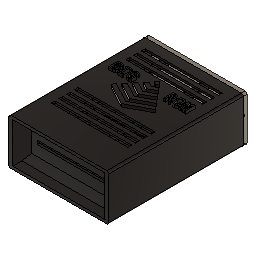
case (Autodesk Fusion 360 design; units mm, degrees)
Autodesk Fusion 360 part; units mm, degrees
note: some values were not read from the file. Chosen so that the rebuilt part matches the saved one: which bodies a step acts on.
(part 1 of 3)
sketch "Schizzo1" plane through (0, 0, 0) normal (0, 0, 1) x (1, 0, 0)
  line L0 (0, 0) -> (52, 0)
  line L1 (52, 0) -> (52, 70)
  line L2 (52, 70) -> (0, 70)
  line L3 (0, 70) -> (0, 0)
  dimension "d1" = 52
  dimension "d2" = 70
  constraint horizontal L0
  constraint vertical L1
  constraint horizontal L2
  constraint vertical L3
  constraint coincident L0.start L3.end
  measures "d1" distance of L0.start L0.end
  measures "d2" distance of L0.start L2.end
extrude "Estrusione1" add sketch "Schizzo1" along normal blind 24 makes body 1
sketch "Schizzo2" plane through (0, 0, 0) normal (0, -1, 0) x (1, 0, 0)
  line L0 (0, 0) -> (52, 0)
  line L1 (52, 0) -> (52, 24)
  line L2 (52, 24) -> (0, 24)
  line L3 (0, 24) -> (0, 0)
  line L4 (2, 22.5) -> (50, 22.5)
  line L5 (50, 22.5) -> (50, 1.5)
  line L6 (50, 1.5) -> (2, 1.5)
  line L7 (2, 1.5) -> (2, 22.5)
  dimension "d5" = 2
  dimension "d6" = 1.5
  dimension "d7" = 1.5
  dimension "d8" = 2
  constraint horizontal L4
  constraint vertical L5
  constraint horizontal L6
  constraint vertical L7
  measures "d5" horizontal distance of L2.end L4.start
  measures "d6" vertical distance of L2.end L4.start
  measures "d7" vertical distance of L0.start L6.end
  measures "d8" horizontal distance of L0.end L5.end
extrude "Estrusione2" cut sketch "Schizzo2" against normal blind 9.8 contours L4 L5 L6 L7 bodies 1
sketch "Schizzo3" plane through (0, 70, 0) normal (0, 1, 0) x (-1, 0, 0)
  line L0 (-52, 0) -> (0, 0)
  line L1 (0, 0) -> (0, 24)
  line L2 (0, 24) -> (-52, 24)
  line L3 (-52, 24) -> (-52, 0)
  line L4 (-48, 1) -> (-48, 8)
  line L5 (-48, 8) -> (-50.25, 8)
  line L6 (-50.25, 8) -> (-50.25, 9.7)
  line L7 (-50.25, 9.7) -> (-48, 9.7)
  line L8 (-48, 9.7) -> (-48, 23)
  line L9 (-48, 23) -> (-4, 23)
  line L10 (-4, 23) -> (-4, 9.7)
  line L11 (-4, 9.7) -> (-1.75, 9.7)
  line L12 (-1.75, 9.7) -> (-1.75, 8)
  line L13 (-1.75, 8) -> (-4, 8)
  line L14 (-4, 8) -> (-4, 1)
  line L15 (-4, 1) -> (-48, 1)
  dimension "d11" = 2.25
  dimension "d12" = 1.7
  dimension "d13" = 2.25
  dimension "d14" = 1
  dimension "d15" = 4
  dimension "d16" = 4
  dimension "d17" = 1
  dimension "d62" = 8
  constraint vertical L4
  constraint perpendicular L4 L5
  constraint perpendicular L5 L6
  constraint perpendicular L6 L7
  constraint perpendicular L7 L8
  constraint perpendicular L6 L9
  constraint perpendicular L9 L10
  constraint perpendicular L10 L11
  constraint perpendicular L11 L12
  constraint perpendicular L12 L13
  constraint perpendicular L13 L14
  constraint perpendicular L4 L15
  constraint equal L8 L10
  constraint equal L5 L7
  constraint equal L11 L13
  constraint equal L6 L12
  measures "d11" distance of L4.end L5.end
  measures "d12" distance of L5.end L6.end
  measures "d13" distance of L10.end L11.end
  measures "d14" vertical distance of L2.end L8.end
  measures "d15" horizontal distance of L0.start L4.start
  measures "d16" horizontal distance of L0.end L14.end
  measures "d17" vertical distance of L0.end L14.end
  measures "d62" vertical distance of L0.start L4.end
extrude "Estrusione3" cut sketch "Schizzo3" against normal blind 59 contours L4 L5 L6 L7 L8 L9 L10 L11 L12 L13 L14 L15 bodies 1
sketch "Schizzo4" plane through (0, 11, 0) normal (0, 1, 0) x (-1, 0, 0)
  line L0 (-4, 1) -> (-4, 8)
  line L1 (-4, 8) -> (-1.75, 8)
  line L2 (-1.75, 8) -> (-1.75, 9.7)
  line L3 (-1.75, 9.7) -> (-4, 9.7)
  line L4 (-4, 9.7) -> (-4, 23)
  line L5 (-4, 23) -> (-48, 23)
  line L6 (-48, 23) -> (-48, 9.7)
  line L7 (-48, 9.7) -> (-50.25, 9.7)
  line L8 (-50.25, 9.7) -> (-50.25, 8)
  line L9 (-50.25, 8) -> (-48, 8)
  line L10 (-48, 8) -> (-48, 1)
  line L11 (-48, 1) -> (-4, 1)
  line L12 (-47, 9.85) -> (-5, 9.85)
  line L13 (-5, 9.85) -> (-5, 7.85)
  line L14 (-5, 7.85) -> (-47, 7.85)
  line L15 (-47, 7.85) -> (-47, 9.85)
  line L16 (-26, 23) -> (-26, 1) construction
  line L17 (-50.25, 8.85) -> (-1.75, 8.85) construction
  dimension "d20" = 42
  dimension "d21" = 2
  constraint horizontal L12
  constraint vertical L13
  constraint horizontal L14
  constraint vertical L15
  constraint midpoint L5 L16.start
  constraint midpoint L11 L16.end
  constraint midpoint L8 L17.start
  constraint midpoint L2 L17.end
  constraint symmetric L13.end L14.end L16
  constraint symmetric L12.start L14.end L17
  measures "d20" distance of L12.start L12.end
  measures "d21" distance of L12.start L14.end
extrude "Estrusione4" cut sketch "Schizzo4" against normal through all contours L12 L13 L14 L15 bodies 1
sketch "Schizzo5" plane through (0, 0, 24) normal (0, 0, 1) x (-1, 0, 0)
  line L0 (0, -70) -> (0, 0)
  line L1 (0, 0) -> (-52, 0)
  line L2 (-52, -70) -> (0, -70)
  line L3 (-6, -55) -> (-46, -55)
  line L4 (-6, -30) -> (-46, -30)
  line L5 (-6, -55) -> (-6, -57)
  line L6 (-6, -57) -> (-46, -57)
  line L7 (-46, -57) -> (-46, -55)
  line L8 (-6, -30) -> (-6, -28)
  line L9 (-6, -28) -> (-46, -28)
  line L10 (-46, -28) -> (-46, -30)
  line L11 (-6, -59) -> (-46, -59)
  line L12 (-46, -59) -> (-46, -61)
  line L13 (-46, -61) -> (-6, -61)
  line L14 (-6, -61) -> (-6, -59)
  line L15 (-6, -63) -> (-46, -63)
  line L16 (-46, -63) -> (-46, -65)
  line L17 (-46, -65) -> (-6, -65)
  line L18 (-6, -65) -> (-6, -63)
  line L19 (-6, -26) -> (-46, -26)
  line L20 (-46, -26) -> (-46, -24)
  line L21 (-46, -24) -> (-6, -24)
  line L22 (-6, -24) -> (-6, -26)
  line L23 (-6, -22) -> (-46, -22)
  line L24 (-46, -22) -> (-46, -20)
  line L25 (-46, -20) -> (-6, -20)
  line L26 (-6, -20) -> (-6, -22)
  line L27 (-6, -18) -> (-46, -18)
  line L28 (-46, -18) -> (-46, -16)
  line L29 (-46, -16) -> (-6, -16)
  line L30 (-6, -16) -> (-6, -18)
  dimension "d34" = 25
  dimension "d146" = 40
  dimension "d147" = 2
  dimension "d148" = 40
  dimension "d149" = 2
  dimension "d150" = 40
  dimension "d151" = 2
  dimension "d152" = 40
  dimension "d153" = 2
  dimension "d154" = 40
  dimension "d155" = 2
  dimension "d156" = 2
  dimension "d157" = 2
  dimension "d158" = 2
  dimension "d159" = 5
  dimension "d160" = 6
  dimension "d162" = 40
  dimension "d163" = 40
  dimension "d164" = 2
  dimension "d165" = 2
  dimension "d166" = 2
  dimension "d167" = 6
  dimension "d168" = 16
  constraint horizontal L4
  constraint equal L3 L4
  constraint perpendicular L3 L5
  constraint perpendicular L5 L6
  constraint perpendicular L4 L8
  constraint perpendicular L8 L9
  constraint horizontal L11
  constraint vertical L12
  constraint horizontal L13
  constraint vertical L14
  constraint horizontal L15
  constraint vertical L16
  constraint horizontal L17
  constraint vertical L18
  constraint horizontal L19
  constraint vertical L20
  constraint horizontal L21
  constraint vertical L22
  constraint horizontal L23
  constraint vertical L24
  constraint horizontal L25
  constraint vertical L26
  constraint horizontal L27
  constraint vertical L28
  constraint horizontal L29
  constraint vertical L30
  constraint equal L4 L9
  constraint vertical L25.end L27.start
  constraint vertical L21.end L23.start
  measures "d34" distance of L3.start L4.start
  measures "d146" distance of L11.start L11.end
  measures "d147" distance of L11.start L13.end
  measures "d148" distance of L15.start L15.end
  measures "d149" distance of L15.start L17.end
  measures "d150" distance of L19.start L19.end
  measures "d151" distance of L19.start L21.end
  measures "d152" distance of L23.start L23.end
  measures "d153" distance of L23.start L25.end
  measures "d154" distance of L27.start L27.end
  measures "d155" distance of L27.start L29.end
  measures "d156" distance of L3.start L5.end
  measures "d157" distance of L5.end L11.start
  measures "d158" distance of L13.end L15.start
  measures "d159" vertical distance of L0.start L17.end
  measures "d160" horizontal distance of L0.start L17.end
  measures "d162" distance of L5.end L6.end
  measures "d163" distance of L3.start L3.end
  measures "d164" distance of L8.end L19.start
  measures "d165" distance of L21.end L23.start
  measures "d166" distance of L25.end L27.start
  measures "d167" horizontal distance of L0.end L29.end
  measures "d168" vertical distance of L1.end L28.end
extrude "Estrusione5" cut sketch "Schizzo5" against normal blind 2 bodies 1
sketch "Schizzo6" plane through (0, 70, 0) normal (0, 1, 0) x (-1, 0, 0)
  line L0 (-1.75, 8) -> (-4, 8)
  line L1 (-4, 8) -> (-4, 1)
  line L2 (-4, 1) -> (-48, 1)
  line L3 (-48, 1) -> (-48, 8)
  line L4 (-48, 8) -> (-50.25, 8)
  line L5 (-50.25, 8) -> (-50.25, 9.7)
  line L6 (-50.25, 9.7) -> (-48, 9.7)
  line L7 (-48, 9.7) -> (-48, 23)
  line L8 (-48, 23) -> (-4, 23)
  line L9 (-4, 23) -> (-4, 9.7)
  line L10 (-4, 9.7) -> (-1.75, 9.7)
  line L11 (-1.75, 9.7) -> (-1.75, 8)
  line L12 (-52, 0) -> (0, 0)
  line L13 (0, 0) -> (0, 24)
  line L14 (0, 24) -> (-52, 24)
  line L15 (-52, 24) -> (-52, 0)
  circle A0 centre (-50, 12.7) radius 1
  circle A1 centre (-2, 12.7) radius 1
  dimension "d44" = 2
  dimension "d45" = 2
  dimension "d46" = 2
  dimension "d47" = 2
  dimension "d121" = 3
  constraint horizontal A0.centre A1.centre
  measures "d44" horizontal distance of L14.end A0.centre
  measures "d45" diameter of A0
  measures "d46" diameter of A1
  measures "d47" horizontal distance of L13.end A1.centre
  measures "d121" vertical distance of L5.end A0.centre
hole "Foratura1" at (50, 70, 12.7) at (2, 70, 12.7) direction (0, -1, 0) diameter 1.3 depth 20 tip angle 118 bodies 1
sketch "Schizzo7" plane through (0, 0, 1) normal (0, 0, 1) x (-1, 0, 0)
  line L0 (-48, -70) -> (-4, -70)
  line L1 (-4, -70) -> (-4, -11)
  line L2 (-4, -11) -> (-48, -11)
  line L3 (-48, -11) -> (-48, -70)
  line L4 (-14, -11) -> (-14, -31)
  line L5 (-14, -31) -> (-4, -31)
  line L6 (-4, -46) -> (-14, -46)
  line L7 (-14, -46) -> (-14, -70)
  line L8 (-17, -70) -> (-17, -46)
  line L9 (-17, -46) -> (-35, -46)
  line L10 (-35, -46) -> (-35, -70)
  line L11 (-38, -70) -> (-38, -46)
  line L12 (-38, -46) -> (-48, -46)
  line L13 (-48, -31) -> (-38, -31)
  line L14 (-38, -31) -> (-38, -11)
  line L15 (-38, -11) -> (-35, -11)
  line L16 (-35, -31) -> (-17, -31)
  line L17 (-17, -31) -> (-17, -11)
  line L18 (-35, -31) -> (-35, -11)
  line L19 (-4, -46) -> (-4, -31)
  line L20 (-48, -46) -> (-48, -31)
  line L21 (-14, -11) -> (-17, -11)
  line L22 (-14, -70) -> (-17, -70)
  line L23 (-35, -70) -> (-38, -70)
  dimension "d52" = 20
  dimension "d53" = 3
  dimension "d54" = 10
  dimension "d55" = 15
  constraint coincident L2 L4.start
  constraint perpendicular L2 L4
  constraint coincident L1 L5.end
  constraint perpendicular L1 L5
  constraint coincident L1 L6.start
  constraint perpendicular L1 L6
  constraint coincident L0 L7.end
  constraint perpendicular L0 L7
  constraint coincident L0 L8.start
  constraint perpendicular L0 L8
  constraint perpendicular L8 L9
  constraint coincident L0 L10.end
  constraint perpendicular L0 L10
  constraint coincident L0 L11.start
  constraint perpendicular L0 L11
  constraint coincident L3 L12.end
  constraint perpendicular L3 L12
  constraint coincident L3 L13.start
  constraint perpendicular L3 L13
  constraint coincident L2 L14.end
  constraint perpendicular L2 L14
  constraint coincident L2 L15.end
  constraint perpendicular L3 L15
  constraint parallel L15 L16
  constraint coincident L2 L17.end
  constraint perpendicular L16 L17
  constraint perpendicular L15 L18
  constraint equal L15 L21
  constraint equal L22 L23
  constraint equal L21 L22
  constraint equal L19 L20
  constraint equal L14 L18
  constraint equal L4 L18
  constraint equal L7 L8
  constraint equal L5 L6
  constraint equal L9 L16
  constraint equal L5 L13
  measures "d52" distance of L4.start L4.end
  measures "d53" distance of L4.start L17.end
  measures "d54" distance of L4.end L5.end
  measures "d55" distance of L5.end L6.start
extrude "Estrusione6" add sketch "Schizzo7" along normal blind 1.5 contours L0 L1 L2 L3 L4 L5 L6 L7 L8 L9 L10 L11 L12 L13 L14 L15 L16 L17 L18 L19 L20 L21 L22 L23 bodies 1
ref_plane "Piano di lavoro2" through (0, 0, 23) normal (0, 0, 1) x (1, 0, 0)
sketch "Schizzo10" plane through (0, 0, 23) normal (0, 0, 1) x (1, 0, 0)
  line L0 (38, 70) -> (38, 50)
  line L1 (38, 50) -> (48, 50)
  line L2 (48, 50) -> (48, 35)
  line L3 (48, 35) -> (38, 35)
  line L4 (38, 35) -> (38, 11)
  line L5 (38, 11) -> (35, 11)
  line L6 (35, 11) -> (35, 35)
  line L7 (35, 35) -> (17, 35)
  line L8 (17, 35) -> (17, 11)
  line L9 (17, 11) -> (14, 11)
  line L10 (14, 11) -> (14, 35)
  line L11 (14, 35) -> (4, 35)
  line L12 (4, 35) -> (4, 50)
  line L13 (4, 50) -> (14, 50)
  line L14 (14, 50) -> (14, 70)
  line L15 (14, 70) -> (17, 70)
  line L16 (17, 70) -> (17, 50)
  line L17 (17, 50) -> (35, 50)
  line L18 (35, 50) -> (35, 70)
  line L19 (35, 70) -> (38, 70)
  line L20 (48, 70) -> (4, 70)
  line L21 (48, 11) -> (4, 11)
  dimension "d65" = 3
  dimension "d66" = 15
  dimension "d67" = 20
  dimension "d68" = 10
  constraint vertical L0
  constraint perpendicular L0 L1
  constraint perpendicular L1 L2
  constraint perpendicular L2 L3
  constraint perpendicular L1 L4
  constraint perpendicular L4 L5
  constraint perpendicular L5 L6
  constraint perpendicular L6 L7
  constraint perpendicular L5 L8
  constraint perpendicular L8 L9
  constraint perpendicular L9 L10
  constraint perpendicular L10 L11
  constraint perpendicular L11 L12
  constraint perpendicular L12 L13
  constraint perpendicular L11 L14
  constraint perpendicular L14 L15
  constraint perpendicular L15 L16
  constraint perpendicular L16 L17
  constraint perpendicular L15 L18
  constraint perpendicular L0 L19
  constraint equal L5 L19
  constraint equal L9 L15
  constraint equal L5 L9
  constraint equal L0 L18
  constraint equal L16 L18
  constraint equal L14 L16
  constraint equal L8 L10
  constraint equal L4 L6
  constraint equal L1 L3
  constraint equal L7 L17
  constraint coincident L18.end L20
  constraint coincident L5.end L21
  constraint equal L1 L13
  constraint coincident L8.end L21
  constraint vertical L11.end L21.end
  constraint vertical L2.end L21.start
  measures "d65" distance of L0.start L18.end
  measures "d66" distance of L1.end L2.end
  measures "d67" distance of L0.start L0.end
  measures "d68" distance of L0.end L1.end
extrude "Estrusione7" add sketch "Schizzo10" against normal blind 1.5 contours L0 L1 L2 L3 L4 L5 L6 L7 L8 L9 L10 L11 L12 L13 L14 L15 L16 L17 L18 L19 L20 L21 bodies 1
sketch "Schizzo11" plane through (0, 0, 24) normal (0, 0, 1) x (-1, 0, 0)
  line L0 (-6, -30) -> (-46, -30)
  line L1 (-46, -55) -> (-6, -55)
  line L2 (0, -70) -> (0, 0)
  line L3 (0, 0) -> (-52, 0)
  line L4 (-52, 0) -> (-52, -70)
  line L5 (-52, -70) -> (0, -70)
  line L6 (-6, -50.9797) -> (-7.5273, -50.9797)
  spline S0 degree 2 poles (-7.5273, -50.9797) (-8.4582, -50.9797) (-8.8924, -50.6722) knots 0 0 0 1 1 1
  spline S1 degree 2 poles (-8.8924, -50.6722) (-9.3266, -50.3647) (-9.3266, -49.685) knots 0 0 0 1 1 1
  spline S2 degree 2 poles (-9.3266, -49.685) (-9.3266, -49.2344) (-9.0486, -48.9336) knots 0 0 0 1 1 1
  spline S3 degree 2 poles (-9.4618, -47.4715) (-9.4618, -46.7868) (-9.0172, -46.3934) knots 0 0 0 1 1 1
  spline S4 degree 2 poles (-9.0172, -46.3934) (-8.5725, -46) (-7.8154, -46) knots 0 0 0 1 1 1
  line L7 (-7.8154, -46) -> (-6, -46)
  line L8 (-6, -46) -> (-6, -50.9797)
  line L9 (-6.7552, -48.9277) -> (-7.6187, -48.9277)
  spline S5 degree 2 poles (-7.6187, -48.9277) (-8.1089, -48.9277) (-8.3219, -49.0924) knots 0 0 0 1 1 1
  spline S6 degree 2 poles (-8.3219, -49.0924) (-8.535, -49.2572) (-8.535, -49.6441) knots 0 0 0 1 1 1
  spline S7 degree 2 poles (-8.535, -49.6441) (-8.535, -50.0046) (-8.306, -50.161) knots 0 0 0 1 1 1
  spline S8 degree 2 poles (-8.306, -50.161) (-8.077, -50.3175) (-7.5529, -50.3175) knots 0 0 0 1 1 1
  line L10 (-7.5529, -50.3175) -> (-6.7552, -50.3175)
  line L11 (-6.7552, -50.3175) -> (-6.7552, -48.9277)
  line L12 (-6.7552, -48.2654) -> (-6.7552, -46.6622)
  line L13 (-6.7552, -46.6622) -> (-7.7043, -46.6622)
  spline S9 degree 2 poles (-7.7043, -46.6622) (-8.6702, -46.6622) (-8.6702, -47.4967) knots 0 0 0 1 1 1
  spline S10 degree 2 poles (-8.6702, -47.4967) (-8.6702, -48.2654) (-7.6611, -48.2654) knots 0 0 0 1 1 1
  line L14 (-7.6611, -48.2654) -> (-6.7552, -48.2654)
  line L15 (-13.1262, -46) -> (-10.4187, -46)
  line L16 (-10.4187, -46) -> (-10.4187, -46.5376)
  line L17 (-10.4187, -46.5376) -> (-11.3966, -46.6039)
  line L18 (-11.3966, -46.6039) -> (-11.3966, -50.3747)
  line L19 (-11.3966, -50.3747) -> (-10.4187, -50.441)
  line L20 (-10.4187, -50.441) -> (-10.4187, -50.9797)
  line L21 (-10.4187, -50.9797) -> (-13.1262, -50.9797)
  line L22 (-13.1262, -50.9797) -> (-13.1262, -50.4413)
  line L23 (-13.1262, -50.4413) -> (-12.1517, -50.3751)
  line L24 (-12.1517, -50.3751) -> (-12.1517, -46.6036)
  line L25 (-12.1517, -46.6036) -> (-13.1262, -46.5373)
  line L26 (-13.1262, -46.5373) -> (-13.1262, -46)
  line L27 (-16.0196, -48.6944) -> (-17.5571, -48.6944)
  line L28 (-17.5571, -48.6944) -> (-17.5571, -46.2033)
  spline S11 degree 2 poles (-17.5571, -46.2033) (-16.8532, -45.9324) (-16.0939, -45.9324) knots 0 0 0 1 1 1
  spline S12 degree 2 poles (-16.0939, -45.9324) (-15.19, -45.9324) (-14.6849, -46.6156) knots 0 0 0 1 1 1
  spline S13 degree 2 poles (-14.6849, -46.6156) (-14.1799, -47.2988) (-14.1799, -48.4965) knots 0 0 0 1 1 1
  spline S14 degree 2 poles (-14.1799, -48.4965) (-14.1799, -49.6843) (-14.7346, -50.3675) knots 0 0 0 1 1 1
  spline S15 degree 2 poles (-14.7346, -50.3675) (-15.2893, -51.0507) (-16.2629, -51.0507) knots 0 0 0 1 1 1
  spline S16 degree 2 poles (-16.2629, -51.0507) (-16.9168, -51.0507) (-17.4809, -50.7257) knots 0 0 0 1 1 1
  line L29 (-17.4809, -50.7257) -> (-17.2047, -50.0935)
  spline S17 degree 2 poles (-17.2047, -50.0935) (-16.669, -50.3719) (-16.2445, -50.3719) knots 0 0 0 1 1 1
  spline S18 degree 2 poles (-16.2445, -50.3719) (-15.647, -50.3719) (-15.3092, -49.8807) knots 0 0 0 1 1 1
  spline S19 degree 2 poles (-15.3092, -49.8807) (-14.9715, -49.3894) (-14.9715, -48.4915) knots 0 0 0 1 1 1
  spline S20 degree 2 poles (-14.9715, -48.4915) (-14.9715, -46.6112) (-16.2022, -46.6112) knots 0 0 0 1 1 1
  spline S21 degree 2 poles (-16.2022, -46.6112) (-16.5151, -46.6112) (-16.802, -46.6906) knots 0 0 0 1 1 1
  line L30 (-16.802, -46.6906) -> (-16.802, -48.0156)
  line L31 (-16.802, -48.0156) -> (-16.0196, -48.0156)
  line L32 (-16.0196, -48.0156) -> (-16.0196, -48.6944)
  spline S22 degree 2 poles (-9.0486, -48.9336) (-8.8398, -48.7075) (-8.5566, -48.6203) knots 0 0 0 0.751565 0.751565 0.751565
  spline S23 degree 2 poles (-8.5566, -48.6203) (-9.4618, -48.3879) (-9.4618, -47.4715) knots 0.093077 0.093077 0.093077 1 1 1
  line L33 (-35.2961, -47.9983) -> (-35.2961, -46)
  line L34 (-35.2961, -46) -> (-34.5409, -46)
  line L35 (-34.5409, -46) -> (-34.5409, -50.9797)
  line L36 (-34.5409, -50.9797) -> (-35.792, -50.9797)
  spline S24 degree 2 poles (-35.792, -50.9797) (-37.5869, -50.9797) (-37.5869, -49.5355) knots 0 0 0 1 1 1
  spline S25 degree 2 poles (-37.5869, -49.5355) (-37.5869, -48.5363) (-36.6274, -48.1996) knots 0 0 0 1 1 1
  line L37 (-36.6274, -48.1996) -> (-37.9461, -46)
  line L38 (-37.9461, -46) -> (-37.1091, -46)
  line L39 (-37.1091, -46) -> (-35.9453, -47.9983)
  line L40 (-35.9453, -47.9983) -> (-35.2961, -47.9983)
  line L41 (-35.2961, -48.6606) -> (-35.7655, -48.6606)
  spline S26 degree 2 poles (-35.7655, -48.6606) (-36.305, -48.6606) (-36.5502, -48.8613) knots 0 0 0 1 1 1
  spline S27 degree 2 poles (-36.5502, -48.8613) (-36.7953, -49.0621) (-36.7953, -49.5072) knots 0 0 0 1 1 1
  spline S28 degree 2 poles (-36.7953, -49.5072) (-36.7953, -49.9402) (-36.5531, -50.1288) knots 0 0 0 1 1 1
  spline S29 degree 2 poles (-36.5531, -50.1288) (-36.311, -50.3175) (-35.749, -50.3175) knots 0 0 0 1 1 1
  line L42 (-35.749, -50.3175) -> (-35.2961, -50.3175)
  line L43 (-35.2961, -50.3175) -> (-35.2961, -48.6606)
  spline S30 degree 2 poles (-40.1538, -45.9324) (-38.3215, -45.9324) (-38.3215, -48.5032) knots 0 0 0 1 1 1
  spline S31 degree 2 poles (-38.3215, -48.5032) (-38.3215, -51.0575) (-40.1604, -51.0575) knots 0 0 0 1 1 1
  spline S32 degree 2 poles (-40.1604, -51.0575) (-41.0466, -51.0575) (-41.5164, -50.385) knots 0 0 0 1 1 1
  spline S33 degree 2 poles (-41.5164, -50.385) (-41.9861, -49.7124) (-41.9861, -48.4966) knots 0 0 0 1 1 1
  spline S34 degree 2 poles (-41.9861, -48.4966) (-41.9861, -47.2795) (-41.5117, -46.606) knots 0 0 0 1 1 1
  spline S35 degree 2 poles (-41.5117, -46.606) (-41.0372, -45.9324) (-40.1538, -45.9324) knots 0 0 0 1 1 1
  spline S36 degree 2 poles (-40.1538, -46.6112) (-40.6881, -46.6112) (-40.9413, -47.0666) knots 0 0 0 1 1 1
  spline S37 degree 2 poles (-40.9413, -47.0666) (-41.1945, -47.5219) (-41.1945, -48.4983) knots 0 0 0 1 1 1
  spline S38 degree 2 poles (-41.1945, -48.4983) (-41.1945, -49.483) (-40.938, -49.9308) knots 0 0 0 1 1 1
  spline S39 degree 2 poles (-40.938, -49.9308) (-40.6815, -50.3786) (-40.1604, -50.3786) knots 0 0 0 1 1 1
  spline S40 degree 2 poles (-40.1604, -50.3786) (-39.1131, -50.3786) (-39.1131, -48.4983) knots 0 0 0 1 1 1
  spline S41 degree 2 poles (-39.1131, -48.4983) (-39.1131, -46.6112) (-40.1538, -46.6112) knots 0 0 0 1 1 1
  line L44 (-43.9423, -46) -> (-43.1615, -49.596)
  line L45 (-43.1806, -48.9646) -> (-43.1806, -46)
  line L46 (-43.1806, -46) -> (-42.5382, -46)
  line L47 (-42.5382, -46) -> (-42.5382, -50.9797)
  line L48 (-42.5382, -50.9797) -> (-43.4818, -50.9797)
  line L49 (-43.4818, -50.9797) -> (-44.2572, -47.2526)
  line L50 (-44.2572, -47.2526) -> (-45.0388, -50.9797)
  line L51 (-45.0388, -50.9797) -> (-46, -50.9797)
  line L52 (-46, -50.9797) -> (-46, -46)
  line L53 (-46, -46) -> (-45.3576, -46)
  line L54 (-45.3576, -46) -> (-45.3576, -49.0077)
  line L55 (-45.3766, -49.6687) -> (-44.5647, -46)
  line L56 (-44.5647, -46) -> (-43.9423, -46)
  spline S42 degree 2 poles (-43.1615, -49.596) (-43.1806, -49.2202) (-43.1806, -48.9646) knots 0.433911 0.433911 0.433911 1 1 1
  spline S43 degree 2 poles (-45.3576, -49.0077) (-45.3576, -49.2263) (-45.3766, -49.6687) knots 0 0 0 0.640385 0.640385 0.640385
  line L57 (-46, -28) -> (-6, -28)
  line L58 (-6, -28) -> (-6, -30)
  line L59 (-46, -30) -> (-46, -28)
  line L60 (-46, -57) -> (-46, -55)
  line L61 (-6, -55) -> (-6, -57)
  line L62 (-6, -57) -> (-46, -57)
  line L63 (-46, -18) -> (-46, -16)
  line L64 (-46, -16) -> (-6, -16)
  line L65 (-6, -16) -> (-6, -18)
  line L66 (-6, -18) -> (-46, -18)
  line L67 (-46, -22) -> (-46, -20)
  line L68 (-46, -20) -> (-6, -20)
  line L69 (-6, -20) -> (-6, -22)
  line L70 (-6, -22) -> (-46, -22)
  line L71 (-46, -59) -> (-6, -59)
  line L72 (-6, -59) -> (-6, -61)
  line L73 (-6, -61) -> (-46, -61)
  line L74 (-46, -61) -> (-46, -59)
  line L75 (-46, -26) -> (-46, -24)
  line L76 (-46, -24) -> (-6, -24)
  line L77 (-6, -24) -> (-6, -26)
  line L78 (-6, -26) -> (-46, -26)
  line L79 (-46, -63) -> (-6, -63)
  line L80 (-6, -63) -> (-6, -65)
  line L81 (-6, -65) -> (-46, -65)
  line L82 (-46, -65) -> (-46, -63)
extrude "Estrusione1'" add sketch "Schizzo11" along normal blind 1.5 separate body contours L6 S0 S1 S2 S3 S4 L7 L8 S22 S23 | L15 L16 L17 L18 L19 L20 L21 L22 L23 L24 L25 L26 | L27 L28 S11 S12 S13 S14 S15 S16 L29 S17 S18 S19 S20 S21 L30 L31 L32 | L33 L34 L35 L36 S24 S25 L37 L38 L39 L40 | S30 S31 S32 S33 S34 S35 | L44 L45 L46 L47 L48 L49 L50 L51 L52 L53 L54 L55 L56 S42 S43 makes body 2 at (11.9, 47.8609, 24) makes body 3 at (17.3054, 47.6377, 24) makes body 4 at (43.0605, 50.5185, 24) makes body 5 at (6.2517, 48.415, 24) makes body 6 at (38.6059, 48.8805, 24) makes body 7 at (34.7926, 48.5468, 24) in component "Componente_Testo"
sketch "Schizzo12" plane through (0, 0, 24) normal (0, 0, 1) x (-1, 0, 0)
  line L0 (-6, -30) -> (-46, -30)
  line L1 (-46, -55) -> (-6, -55)
  line L2 (0, -70) -> (0, 0)
  line L3 (0, 0) -> (-52, 0)
  line L4 (-52, 0) -> (-52, -70)
  line L5 (-52, -70) -> (0, -70)
  spline S0 degree 3 poles (-25.8442, -38.9932) (-25.6519, -39.0542) (-25.2683, -39.375) (-24.4958, -39.8248) knots 0 0 0 0 1 1 1 1
  line L6 (-25.8442, -38.9932) -> (-25.6519, -39.0542) construction
  line L7 (-25.6519, -39.0542) -> (-25.2683, -39.375) construction
  line L8 (-25.2683, -39.375) -> (-24.4958, -39.8248) construction
  spline S1 degree 3 poles (-24.4958, -39.8248) (-23.9962, -40.1158) (-23.6534, -40.3101) (-22.8266, -40.7709) knots 0 0 0 0 1 1 1 1
  line L9 (-24.4958, -39.8248) -> (-23.9962, -40.1158) construction
  line L10 (-23.9962, -40.1158) -> (-23.6534, -40.3101) construction
  line L11 (-23.6534, -40.3101) -> (-22.8266, -40.7709) construction
  spline S2 degree 3 poles (-22.8266, -40.7709) (-20.957, -41.8131) (-19.8024, -42.4728) (-19.2156, -42.8342) knots 0 0 0 0 1 1 1 1
  line L12 (-22.8266, -40.7709) -> (-20.957, -41.8131) construction
  line L13 (-20.957, -41.8131) -> (-19.8024, -42.4728) construction
  line L14 (-19.8024, -42.4728) -> (-19.2156, -42.8342) construction
  spline S3 degree 3 poles (-19.2156, -42.8342) (-19.0296, -42.9487) (-18.8671, -43.0807) (-18.8872, -43.1008) knots 0 0 0 0 1 1 1 1
  line L15 (-19.2156, -42.8342) -> (-19.0296, -42.9487) construction
  line L16 (-19.0296, -42.9487) -> (-18.8671, -43.0807) construction
  line L17 (-18.8671, -43.0807) -> (-18.8872, -43.1008) construction
  spline S4 degree 3 poles (-18.8872, -43.1008) (-18.9205, -43.1341) (-19.4317, -42.875) (-21.4715, -41.7912) knots 0 0 0 0 1 1 1 1
  line L18 (-18.8872, -43.1008) -> (-18.9205, -43.1341) construction
  line L19 (-18.9205, -43.1341) -> (-19.4317, -42.875) construction
  line L20 (-19.4317, -42.875) -> (-21.4715, -41.7912) construction
  spline S5 degree 3 poles (-21.4715, -41.7912) (-23.3012, -40.8189) (-23.623, -40.65) (-24.2975, -40.3075) knots 0 0 0 0 1 1 1 1
  line L21 (-21.4715, -41.7912) -> (-23.3012, -40.8189) construction
  line L22 (-23.3012, -40.8189) -> (-23.623, -40.65) construction
  line L23 (-23.623, -40.65) -> (-24.2975, -40.3075) construction
  spline S6 degree 3 poles (-24.2975, -40.3075) (-25.2513, -39.8233) (-25.8208, -39.5674) (-26.0954, -39.4997) knots 0 0 0 0 1 1 1 1
  line L24 (-24.2975, -40.3075) -> (-25.2513, -39.8233) construction
  line L25 (-25.2513, -39.8233) -> (-25.8208, -39.5674) construction
  line L26 (-25.8208, -39.5674) -> (-26.0954, -39.4997) construction
  spline S7 degree 3 poles (-26.0954, -39.4997) (-26.2199, -39.469) (-26.2449, -39.473) (-26.3442, -39.5398) knots 0 0 0 0 1 1 1 1
  line L27 (-26.0954, -39.4997) -> (-26.2199, -39.469) construction
  line L28 (-26.2199, -39.469) -> (-26.2449, -39.473) construction
  line L29 (-26.2449, -39.473) -> (-26.3442, -39.5398) construction
  spline S8 degree 3 poles (-26.3442, -39.5398) (-26.6301, -39.7321) (-28.7547, -40.9015) (-30.9081, -42.0517) knots 0 0 0 0 1 1 1 1
  line L30 (-26.3442, -39.5398) -> (-26.6301, -39.7321) construction
  line L31 (-26.6301, -39.7321) -> (-28.7547, -40.9015) construction
  line L32 (-28.7547, -40.9015) -> (-30.9081, -42.0517) construction
  spline S9 degree 3 poles (-30.9081, -42.0517) (-32.1515, -42.7159) (-32.7299, -43.0398) (-32.8996, -43.167) knots 0 0 0 0 1 1 1 1
  line L33 (-30.9081, -42.0517) -> (-32.1515, -42.7159) construction
  line L34 (-32.1515, -42.7159) -> (-32.7299, -43.0398) construction
  line L35 (-32.7299, -43.0398) -> (-32.8996, -43.167) construction
  spline S10 degree 3 poles (-32.8996, -43.167) (-33.0006, -43.2428) (-33.1641, -43.2825) (-33.3738, -43.2824) knots 0 0 0 0 1 1 1 1
  line L36 (-32.8996, -43.167) -> (-33.0006, -43.2428) construction
  line L37 (-33.0006, -43.2428) -> (-33.1641, -43.2825) construction
  line L38 (-33.1641, -43.2825) -> (-33.3738, -43.2824) construction
  spline S11 degree 3 poles (-33.3738, -43.2824) (-33.4756, -43.2824) (-33.5643, -43.2769) (-33.5709, -43.2702) knots 0 0 0 0 1 1 1 1
  line L39 (-33.3738, -43.2824) -> (-33.4756, -43.2824) construction
  line L40 (-33.4756, -43.2824) -> (-33.5643, -43.2769) construction
  line L41 (-33.5643, -43.2769) -> (-33.5709, -43.2702) construction
  spline S12 degree 3 poles (-33.5709, -43.2702) (-33.5879, -43.2532) (-33.5041, -43.1688) (-33.3871, -43.0849) knots 0 0 0 0 1 1 1 1
  line L42 (-33.5709, -43.2702) -> (-33.5879, -43.2532) construction
  line L43 (-33.5879, -43.2532) -> (-33.5041, -43.1688) construction
  line L44 (-33.5041, -43.1688) -> (-33.3871, -43.0849) construction
  spline S13 degree 3 poles (-33.3871, -43.0849) (-33.1738, -42.932) (-32.3963, -42.4729) (-30.6437, -41.4653) knots 0 0 0 0 1 1 1 1
  line L45 (-33.3871, -43.0849) -> (-33.1738, -42.932) construction
  line L46 (-33.1738, -42.932) -> (-32.3963, -42.4729) construction
  line L47 (-32.3963, -42.4729) -> (-30.6437, -41.4653) construction
  spline S14 degree 3 poles (-30.6437, -41.4653) (-29.2966, -40.6908) (-28.392, -40.1448) (-27.3301, -39.4655) knots 0 0 0 0 1 1 1 1
  line L48 (-30.6437, -41.4653) -> (-29.2966, -40.6908) construction
  line L49 (-29.2966, -40.6908) -> (-28.392, -40.1448) construction
  line L50 (-28.392, -40.1448) -> (-27.3301, -39.4655) construction
  spline S15 degree 3 poles (-27.3301, -39.4655) (-26.9081, -39.1955) (-26.6858, -39.0537) (-26.6729, -39.0328) knots 0 0 0 0 1 1 1 1
  line L51 (-27.3301, -39.4655) -> (-26.9081, -39.1955) construction
  line L52 (-26.9081, -39.1955) -> (-26.6858, -39.0537) construction
  line L53 (-26.6858, -39.0537) -> (-26.6729, -39.0328) construction
  spline S16 degree 3 poles (-26.6729, -39.0328) (-26.6412, -38.9815) (-26.2253, -38.8722) (-26.1311, -38.9021) knots 0 0 0 0 1 1 1 1
  line L54 (-26.6729, -39.0328) -> (-26.6412, -38.9815) construction
  line L55 (-26.6412, -38.9815) -> (-26.2253, -38.8722) construction
  line L56 (-26.2253, -38.8722) -> (-26.1311, -38.9021) construction
  line L57 (-26.1311, -38.9021) -> (-25.8442, -38.9932)
  spline S17 degree 3 poles (-25.2478, -40.2367) (-24.7615, -40.5097) (-23.5456, -41.1907) (-22.5457, -41.7502) knots 0 0 0 0 1 1 1 1
  line L58 (-25.2478, -40.2367) -> (-24.7615, -40.5097) construction
  line L59 (-24.7615, -40.5097) -> (-23.5456, -41.1907) construction
  line L60 (-23.5456, -41.1907) -> (-22.5457, -41.7502) construction
  spline S18 degree 3 poles (-22.5457, -41.7502) (-20.0466, -43.1487) (-19.588, -43.4111) (-19.4172, -43.54) knots 0 0 0 0 1 1 1 1
  line L61 (-22.5457, -41.7502) -> (-20.0466, -43.1487) construction
  line L62 (-20.0466, -43.1487) -> (-19.588, -43.4111) construction
  line L63 (-19.588, -43.4111) -> (-19.4172, -43.54) construction
  spline S19 degree 3 poles (-19.4172, -43.54) (-19.3369, -43.6007) (-19.3078, -43.6551) (-19.3557, -43.6551) knots 0 0 0 0 1 1 1 1
  line L64 (-19.4172, -43.54) -> (-19.3369, -43.6007) construction
  line L65 (-19.3369, -43.6007) -> (-19.3078, -43.6551) construction
  line L66 (-19.3078, -43.6551) -> (-19.3557, -43.6551) construction
  spline S20 degree 3 poles (-19.3557, -43.6551) (-19.3991, -43.6551) (-19.9707, -43.3788) (-20.6286, -43.0399) knots 0 0 0 0 1 1 1 1
  line L67 (-19.3557, -43.6551) -> (-19.3991, -43.6551) construction
  line L68 (-19.3991, -43.6551) -> (-19.9707, -43.3788) construction
  line L69 (-19.9707, -43.3788) -> (-20.6286, -43.0399) construction
  spline S21 degree 3 poles (-20.6286, -43.0399) (-21.471, -42.6059) (-22.1336, -42.2552) (-24.1838, -41.1585) knots 0 0 0 0 1 1 1 1
  line L70 (-20.6286, -43.0399) -> (-21.471, -42.6059) construction
  line L71 (-21.471, -42.6059) -> (-22.1336, -42.2552) construction
  line L72 (-22.1336, -42.2552) -> (-24.1838, -41.1585) construction
  spline S22 degree 3 poles (-24.1838, -41.1585) (-25.7543, -40.3183) (-25.9548, -40.2153) (-25.9924, -40.2294) knots 0 0 0 0 1 1 1 1
  line L73 (-24.1838, -41.1585) -> (-25.7543, -40.3183) construction
  line L74 (-25.7543, -40.3183) -> (-25.9548, -40.2153) construction
  line L75 (-25.9548, -40.2153) -> (-25.9924, -40.2294) construction
  spline S23 degree 3 poles (-25.9924, -40.2294) (-26.1074, -40.2727) (-30.9223, -42.8641) (-31.8915, -43.4044) knots 0 0 0 0 1 1 1 1
  line L76 (-25.9924, -40.2294) -> (-26.1074, -40.2727) construction
  line L77 (-26.1074, -40.2727) -> (-30.9223, -42.8641) construction
  line L78 (-30.9223, -42.8641) -> (-31.8915, -43.4044) construction
  spline S24 degree 3 poles (-31.8915, -43.4044) (-32.4574, -43.7199) (-32.7291, -43.8369) (-32.8956, -43.8369) knots 0 0 0 0 1 1 1 1
  line L79 (-31.8915, -43.4044) -> (-32.4574, -43.7199) construction
  line L80 (-32.4574, -43.7199) -> (-32.7291, -43.8369) construction
  line L81 (-32.7291, -43.8369) -> (-32.8956, -43.8369) construction
  spline S25 degree 3 poles (-32.8956, -43.8369) (-33.2393, -43.8369) (-32.3281, -43.2549) (-29.0737, -41.3957) knots 0 0 0 0 1 1 1 1
  line L82 (-32.8956, -43.8369) -> (-33.2393, -43.8369) construction
  line L83 (-33.2393, -43.8369) -> (-32.3281, -43.2549) construction
  line L84 (-32.3281, -43.2549) -> (-29.0737, -41.3957) construction
  spline S26 degree 3 poles (-29.0737, -41.3957) (-27.5436, -40.5217) (-26.1587, -39.7383) (-26.1453, -39.7394) knots 0 0 0 0 1 1 1 1
  line L85 (-29.0737, -41.3957) -> (-27.5436, -40.5217) construction
  line L86 (-27.5436, -40.5217) -> (-26.1587, -39.7383) construction
  line L87 (-26.1587, -39.7383) -> (-26.1453, -39.7394) construction
  spline S27 degree 3 poles (-26.1453, -39.7394) (-26.1379, -39.74) (-25.7341, -39.9638) (-25.2478, -40.2367) knots 0 0 0 0 1 1 1 1
  line L88 (-26.1453, -39.7394) -> (-26.1379, -39.74) construction
  line L89 (-26.1379, -39.74) -> (-25.7341, -39.9638) construction
  line L90 (-25.7341, -39.9638) -> (-25.2478, -40.2367) construction
  spline S28 degree 3 poles (-25.6684, -40.8847) (-24.8946, -41.2738) (-24.1823, -41.6626) (-21.9921, -42.8911) knots 0 0 0 0 1 1 1 1
  line L91 (-25.6684, -40.8847) -> (-24.8946, -41.2738) construction
  line L92 (-24.8946, -41.2738) -> (-24.1823, -41.6626) construction
  line L93 (-24.1823, -41.6626) -> (-21.9921, -42.8911) construction
  spline S29 degree 3 poles (-21.9921, -42.8911) (-20.3157, -43.8314) (-19.6592, -44.2034) (-19.6655, -44.2097) knots 0 0 0 0 1 1 1 1
  line L94 (-21.9921, -42.8911) -> (-20.3157, -43.8314) construction
  line L95 (-20.3157, -43.8314) -> (-19.6592, -44.2034) construction
  line L96 (-19.6592, -44.2034) -> (-19.6655, -44.2097) construction
  spline S30 degree 3 poles (-19.6655, -44.2097) (-19.6684, -44.2126) (-19.7465, -44.1937) (-19.8393, -44.1679) knots 0 0 0 0 1 1 1 1
  line L97 (-19.6655, -44.2097) -> (-19.6684, -44.2126) construction
  line L98 (-19.6684, -44.2126) -> (-19.7465, -44.1937) construction
  line L99 (-19.7465, -44.1937) -> (-19.8393, -44.1679) construction
  spline S31 degree 3 poles (-19.8393, -44.1679) (-20.0655, -44.1048) (-20.2698, -44.0115) (-21.1079, -43.5886) knots 0 0 0 0 1 1 1 1
  line L100 (-19.8393, -44.1679) -> (-20.0655, -44.1048) construction
  line L101 (-20.0655, -44.1048) -> (-20.2698, -44.0115) construction
  line L102 (-20.2698, -44.0115) -> (-21.1079, -43.5886) construction
  spline S32 degree 3 poles (-21.1079, -43.5886) (-21.816, -43.2313) (-22.1292, -43.0677) (-23.2894, -42.449) knots 0 0 0 0 1 1 1 1
  line L103 (-21.1079, -43.5886) -> (-21.816, -43.2313) construction
  line L104 (-21.816, -43.2313) -> (-22.1292, -43.0677) construction
  line L105 (-22.1292, -43.0677) -> (-23.2894, -42.449) construction
  spline S33 degree 3 poles (-23.2894, -42.449) (-24.5128, -41.7965) (-25.5758, -41.2513) (-25.8304, -41.1457) knots 0 0 0 0 1 1 1 1
  line L106 (-23.2894, -42.449) -> (-24.5128, -41.7965) construction
  line L107 (-24.5128, -41.7965) -> (-25.5758, -41.2513) construction
  line L108 (-25.5758, -41.2513) -> (-25.8304, -41.1457) construction
  line L109 (-25.8304, -41.1457) -> (-25.9586, -41.0925)
  line L110 (-25.9586, -41.0925) -> (-26.07, -41.1367)
  spline S34 degree 3 poles (-26.07, -41.1367) (-26.3572, -41.2506) (-26.966, -41.5697) (-28.6605, -42.4947) knots 0 0 0 0 1 1 1 1
  line L111 (-26.07, -41.1367) -> (-26.3572, -41.2506) construction
  line L112 (-26.3572, -41.2506) -> (-26.966, -41.5697) construction
  line L113 (-26.966, -41.5697) -> (-28.6605, -42.4947) construction
  spline S35 degree 3 poles (-28.6605, -42.4947) (-31.6741, -44.1397) (-32.4712, -44.5335) (-32.5452, -44.4138) knots 0 0 0 0 1 1 1 1
  line L114 (-28.6605, -42.4947) -> (-31.6741, -44.1397) construction
  line L115 (-31.6741, -44.1397) -> (-32.4712, -44.5335) construction
  line L116 (-32.4712, -44.5335) -> (-32.5452, -44.4138) construction
  spline S36 degree 3 poles (-32.5452, -44.4138) (-32.5829, -44.3528) (-32.0413, -43.9583) (-31.3261, -43.5259) knots 0 0 0 0 1 1 1 1
  line L117 (-32.5452, -44.4138) -> (-32.5829, -44.3528) construction
  line L118 (-32.5829, -44.3528) -> (-32.0413, -43.9583) construction
  line L119 (-32.0413, -43.9583) -> (-31.3261, -43.5259) construction
  spline S37 degree 3 poles (-31.3261, -43.5259) (-31.0673, -43.3693) (-28.6266, -41.9568) (-27.545, -41.3375) knots 0 0 0 0 1 1 1 1
  line L120 (-31.3261, -43.5259) -> (-31.0673, -43.3693) construction
  line L121 (-31.0673, -43.3693) -> (-28.6266, -41.9568) construction
  line L122 (-28.6266, -41.9568) -> (-27.545, -41.3375) construction
  spline S38 degree 3 poles (-27.545, -41.3375) (-27.011, -41.0318) (-26.2981, -40.6676) (-26.2055, -40.6531) knots 0 0 0 0 1 1 1 1
  line L123 (-27.545, -41.3375) -> (-27.011, -41.0318) construction
  line L124 (-27.011, -41.0318) -> (-26.2981, -40.6676) construction
  line L125 (-26.2981, -40.6676) -> (-26.2055, -40.6531) construction
  spline S39 degree 3 poles (-26.2055, -40.6531) (-26.1541, -40.6452) (-26.0872, -40.674) (-25.6684, -40.8847) knots 0 0 0 0 1 1 1 1
  line L126 (-26.2055, -40.6531) -> (-26.1541, -40.6452) construction
  line L127 (-26.1541, -40.6452) -> (-26.0872, -40.674) construction
  line L128 (-26.0872, -40.674) -> (-25.6684, -40.8847) construction
  spline S40 degree 3 poles (-25.7547, -41.6281) (-24.1382, -42.4557) (-20.1279, -44.7536) (-20.2353, -44.7908) knots 0 0 0 0 1 1 1 1
  line L129 (-25.7547, -41.6281) -> (-24.1382, -42.4557) construction
  line L130 (-24.1382, -42.4557) -> (-20.1279, -44.7536) construction
  line L131 (-20.1279, -44.7536) -> (-20.2353, -44.7908) construction
  spline S41 degree 3 poles (-20.2353, -44.7908) (-20.2847, -44.8079) (-21.3533, -44.2887) (-22.4218, -43.7284) knots 0 0 0 0 1 1 1 1
  line L132 (-20.2353, -44.7908) -> (-20.2847, -44.8079) construction
  line L133 (-20.2847, -44.8079) -> (-21.3533, -44.2887) construction
  line L134 (-21.3533, -44.2887) -> (-22.4218, -43.7284) construction
  spline S42 degree 3 poles (-22.4218, -43.7284) (-23.6403, -43.0893) (-25.3489, -42.2424) (-25.7435, -42.0817) knots 0 0 0 0 1 1 1 1
  line L135 (-22.4218, -43.7284) -> (-23.6403, -43.0893) construction
  line L136 (-23.6403, -43.0893) -> (-25.3489, -42.2424) construction
  line L137 (-25.3489, -42.2424) -> (-25.7435, -42.0817) construction
  spline S43 degree 3 poles (-25.7435, -42.0817) (-26.1427, -41.9192) (-26.1595, -41.9219) (-26.6768, -42.2299) knots 0 0 0 0 1 1 1 1
  line L138 (-25.7435, -42.0817) -> (-26.1427, -41.9192) construction
  line L139 (-26.1427, -41.9192) -> (-26.1595, -41.9219) construction
  line L140 (-26.1595, -41.9219) -> (-26.6768, -42.2299) construction
  spline S44 degree 3 poles (-26.6768, -42.2299) (-26.822, -42.3164) (-27.1752, -42.5096) (-27.4618, -42.6594) knots 0 0 0 0 1 1 1 1
  line L141 (-26.6768, -42.2299) -> (-26.822, -42.3164) construction
  line L142 (-26.822, -42.3164) -> (-27.1752, -42.5096) construction
  line L143 (-27.1752, -42.5096) -> (-27.4618, -42.6594) construction
  spline S45 degree 3 poles (-27.4618, -42.6594) (-28.4673, -43.1849) (-29.0331, -43.4832) (-30.0653, -44.032) knots 0 0 0 0 1 1 1 1
  line L144 (-27.4618, -42.6594) -> (-28.4673, -43.1849) construction
  line L145 (-28.4673, -43.1849) -> (-29.0331, -43.4832) construction
  line L146 (-29.0331, -43.4832) -> (-30.0653, -44.032) construction
  spline S46 degree 3 poles (-30.0653, -44.032) (-31.551, -44.822) (-31.9013, -44.9974) (-32.0124, -45.0066) knots 0 0 0 0 1 1 1 1
  line L147 (-30.0653, -44.032) -> (-31.551, -44.822) construction
  line L148 (-31.551, -44.822) -> (-31.9013, -44.9974) construction
  line L149 (-31.9013, -44.9974) -> (-32.0124, -45.0066) construction
  spline S47 degree 3 poles (-32.0124, -45.0066) (-32.1924, -45.0215) (-32.2203, -44.9509) (-32.0857, -44.821) knots 0 0 0 0 1 1 1 1
  line L150 (-32.0124, -45.0066) -> (-32.1924, -45.0215) construction
  line L151 (-32.1924, -45.0215) -> (-32.2203, -44.9509) construction
  line L152 (-32.2203, -44.9509) -> (-32.0857, -44.821) construction
  spline S48 degree 3 poles (-32.0857, -44.821) (-31.9789, -44.718) (-31.8257, -44.6164) (-31.531, -44.4533) knots 0 0 0 0 1 1 1 1
  line L153 (-32.0857, -44.821) -> (-31.9789, -44.718) construction
  line L154 (-31.9789, -44.718) -> (-31.8257, -44.6164) construction
  line L155 (-31.8257, -44.6164) -> (-31.531, -44.4533) construction
  spline S49 degree 3 poles (-31.531, -44.4533) (-30.8602, -44.0821) (-29.9522, -43.5629) (-28.8258, -42.9065) knots 0 0 0 0 1 1 1 1
  line L156 (-31.531, -44.4533) -> (-30.8602, -44.0821) construction
  line L157 (-30.8602, -44.0821) -> (-29.9522, -43.5629) construction
  line L158 (-29.9522, -43.5629) -> (-28.8258, -42.9065) construction
  spline S50 degree 3 poles (-28.8258, -42.9065) (-27.2751, -42.0028) (-26.2505, -41.4412) (-26.1513, -41.4407) knots 0 0 0 0 1 1 1 1
  line L159 (-28.8258, -42.9065) -> (-27.2751, -42.0028) construction
  line L160 (-27.2751, -42.0028) -> (-26.2505, -41.4412) construction
  line L161 (-26.2505, -41.4412) -> (-26.1513, -41.4407) construction
  spline S51 degree 3 poles (-26.1513, -41.4407) (-26.1347, -41.4406) (-25.9562, -41.525) (-25.7547, -41.6281) knots 0 0 0 0 1 1 1 1
  line L162 (-26.1513, -41.4407) -> (-26.1347, -41.4406) construction
  line L163 (-26.1347, -41.4406) -> (-25.9562, -41.525) construction
  line L164 (-25.9562, -41.525) -> (-25.7547, -41.6281) construction
  spline S52 degree 3 poles (-26.0989, -42.2496) (-26.0716, -42.2658) (-25.6403, -42.5044) (-25.1404, -42.7797) knots 0 0 0 0 1 1 1 1
  line L165 (-26.0989, -42.2496) -> (-26.0716, -42.2658) construction
  line L166 (-26.0716, -42.2658) -> (-25.6403, -42.5044) construction
  line L167 (-25.6403, -42.5044) -> (-25.1404, -42.7797) construction
  spline S53 degree 3 poles (-25.1404, -42.7797) (-23.0593, -43.9258) (-22.1452, -44.44) (-21.4321, -44.8656) knots 0 0 0 0 1 1 1 1
  line L168 (-25.1404, -42.7797) -> (-23.0593, -43.9258) construction
  line L169 (-23.0593, -43.9258) -> (-22.1452, -44.44) construction
  line L170 (-22.1452, -44.44) -> (-21.4321, -44.8656) construction
  spline S54 degree 3 poles (-21.4321, -44.8656) (-20.962, -45.1462) (-20.6938, -45.3243) (-20.7414, -45.3243) knots 0 0 0 0 1 1 1 1
  line L171 (-21.4321, -44.8656) -> (-20.962, -45.1462) construction
  line L172 (-20.962, -45.1462) -> (-20.6938, -45.3243) construction
  line L173 (-20.6938, -45.3243) -> (-20.7414, -45.3243) construction
  spline S55 degree 3 poles (-20.7414, -45.3243) (-20.7617, -45.3243) (-21.0956, -45.178) (-21.3762, -45.0462) knots 0 0 0 0 1 1 1 1
  line L174 (-20.7414, -45.3243) -> (-20.7617, -45.3243) construction
  line L175 (-20.7617, -45.3243) -> (-21.0956, -45.178) construction
  line L176 (-21.0956, -45.178) -> (-21.3762, -45.0462) construction
  spline S56 degree 3 poles (-21.3762, -45.0462) (-21.8909, -44.8046) (-23.2296, -44.1232) (-24.6713, -43.369) knots 0 0 0 0 1 1 1 1
  line L177 (-21.3762, -45.0462) -> (-21.8909, -44.8046) construction
  line L178 (-21.8909, -44.8046) -> (-23.2296, -44.1232) construction
  line L179 (-23.2296, -44.1232) -> (-24.6713, -43.369) construction
  spline S57 degree 3 poles (-24.6713, -43.369) (-25.4132, -42.981) (-26.0283, -42.6635) (-26.0382, -42.6635) knots 0 0 0 0 1 1 1 1
  line L180 (-24.6713, -43.369) -> (-25.4132, -42.981) construction
  line L181 (-25.4132, -42.981) -> (-26.0283, -42.6635) construction
  line L182 (-26.0283, -42.6635) -> (-26.0382, -42.6635) construction
  spline S58 degree 3 poles (-26.0382, -42.6635) (-26.0481, -42.6635) (-26.3186, -42.8146) (-26.6394, -42.9993) knots 0 0 0 0 1 1 1 1
  line L183 (-26.0382, -42.6635) -> (-26.0481, -42.6635) construction
  line L184 (-26.0481, -42.6635) -> (-26.3186, -42.8146) construction
  line L185 (-26.3186, -42.8146) -> (-26.6394, -42.9993) construction
  spline S59 degree 3 poles (-26.6394, -42.9993) (-27.5122, -43.5016) (-28.4082, -43.9906) (-29.7926, -44.7199) knots 0 0 0 0 1 1 1 1
  line L186 (-26.6394, -42.9993) -> (-27.5122, -43.5016) construction
  line L187 (-27.5122, -43.5016) -> (-28.4082, -43.9906) construction
  line L188 (-28.4082, -43.9906) -> (-29.7926, -44.7199) construction
  spline S60 degree 3 poles (-29.7926, -44.7199) (-30.6076, -45.1492) (-31.5882, -45.6383) (-31.634, -45.6383) knots 0 0 0 0 1 1 1 1
  line L189 (-29.7926, -44.7199) -> (-30.6076, -45.1492) construction
  line L190 (-30.6076, -45.1492) -> (-31.5882, -45.6383) construction
  line L191 (-31.5882, -45.6383) -> (-31.634, -45.6383) construction
  spline S61 degree 3 poles (-31.634, -45.6383) (-31.7273, -45.6383) (-31.7488, -45.5978) (-31.7027, -45.5086) knots 0 0 0 0 1 1 1 1
  line L192 (-31.634, -45.6383) -> (-31.7273, -45.6383) construction
  line L193 (-31.7273, -45.6383) -> (-31.7488, -45.5978) construction
  line L194 (-31.7488, -45.5978) -> (-31.7027, -45.5086) construction
  spline S62 degree 3 poles (-31.7027, -45.5086) (-31.6637, -45.4332) (-31.4449, -45.2376) (-31.2706, -45.1224) knots 0 0 0 0 1 1 1 1
  line L195 (-31.7027, -45.5086) -> (-31.6637, -45.4332) construction
  line L196 (-31.6637, -45.4332) -> (-31.4449, -45.2376) construction
  line L197 (-31.4449, -45.2376) -> (-31.2706, -45.1224) construction
  spline S63 degree 3 poles (-31.2706, -45.1224) (-31.1267, -45.0273) (-29.1524, -43.8979) (-27.0822, -42.7264) knots 0 0 0 0 1 1 1 1
  line L198 (-31.2706, -45.1224) -> (-31.1267, -45.0273) construction
  line L199 (-31.1267, -45.0273) -> (-29.1524, -43.8979) construction
  line L200 (-29.1524, -43.8979) -> (-27.0822, -42.7264) construction
  spline S64 degree 3 poles (-27.0822, -42.7264) (-26.2105, -42.2331) (-26.1814, -42.217) (-26.1634, -42.2187) knots 0 0 0 0 1 1 1 1
  line L201 (-27.0822, -42.7264) -> (-26.2105, -42.2331) construction
  line L202 (-26.2105, -42.2331) -> (-26.1814, -42.217) construction
  line L203 (-26.1814, -42.217) -> (-26.1634, -42.2187) construction
  spline S65 degree 3 poles (-26.1634, -42.2187) (-26.1552, -42.2194) (-26.1262, -42.2333) (-26.0989, -42.2496) knots 0 0 0 0 1 1 1 1
  line L204 (-26.1634, -42.2187) -> (-26.1552, -42.2194) construction
  line L205 (-26.1552, -42.2194) -> (-26.1262, -42.2333) construction
  line L206 (-26.1262, -42.2333) -> (-26.0989, -42.2496) construction
  spline S66 degree 3 poles (-25.9254, -43.2288) (-25.7276, -43.3116) (-24.7696, -43.7964) (-24.255, -44.074) knots 0 0 0 0 1 1 1 1
  line L207 (-25.9254, -43.2288) -> (-25.7276, -43.3116) construction
  line L208 (-25.7276, -43.3116) -> (-24.7696, -43.7964) construction
  line L209 (-24.7696, -43.7964) -> (-24.255, -44.074) construction
  spline S67 degree 3 poles (-24.255, -44.074) (-23.1067, -44.6936) (-21.9136, -45.3803) (-21.3787, -45.7295) knots 0 0 0 0 1 1 1 1
  line L210 (-24.255, -44.074) -> (-23.1067, -44.6936) construction
  line L211 (-23.1067, -44.6936) -> (-21.9136, -45.3803) construction
  line L212 (-21.9136, -45.3803) -> (-21.3787, -45.7295) construction
  spline S68 degree 3 poles (-21.3787, -45.7295) (-21.0731, -45.929) (-21.0735, -45.9499) (-21.3803, -45.8209) knots 0 0 0 0 1 1 1 1
  line L213 (-21.3787, -45.7295) -> (-21.0731, -45.929) construction
  line L214 (-21.0731, -45.929) -> (-21.0735, -45.9499) construction
  line L215 (-21.0735, -45.9499) -> (-21.3803, -45.8209) construction
  spline S69 degree 3 poles (-21.3803, -45.8209) (-21.8958, -45.6041) (-22.6817, -45.2108) (-24.6799, -44.1698) knots 0 0 0 0 1 1 1 1
  line L216 (-21.3803, -45.8209) -> (-21.8958, -45.6041) construction
  line L217 (-21.8958, -45.6041) -> (-22.6817, -45.2108) construction
  line L218 (-22.6817, -45.2108) -> (-24.6799, -44.1698) construction
  line L219 (-24.6799, -44.1698) -> (-25.9547, -43.5057)
  line L220 (-25.9547, -43.5057) -> (-27.2583, -44.1979)
  spline S70 degree 3 poles (-27.2583, -44.1979) (-29.089, -45.1701) (-29.3871, -45.3261) (-29.9579, -45.6109) knots 0 0 0 0 1 1 1 1
  line L221 (-27.2583, -44.1979) -> (-29.089, -45.1701) construction
  line L222 (-29.089, -45.1701) -> (-29.3871, -45.3261) construction
  line L223 (-29.3871, -45.3261) -> (-29.9579, -45.6109) construction
  spline S71 degree 3 poles (-29.9579, -45.6109) (-30.5456, -45.904) (-30.8225, -46.0254) (-31.0106, -46.0722) knots 0 0 0 0 1 1 1 1
  line L224 (-29.9579, -45.6109) -> (-30.5456, -45.904) construction
  line L225 (-30.5456, -45.904) -> (-30.8225, -46.0254) construction
  line L226 (-30.8225, -46.0254) -> (-31.0106, -46.0722) construction
  spline S72 degree 3 poles (-31.0106, -46.0722) (-31.1382, -46.104) (-31.1486, -46.1044) (-31.1883, -46.0784) knots 0 0 0 0 1 1 1 1
  line L227 (-31.0106, -46.0722) -> (-31.1382, -46.104) construction
  line L228 (-31.1382, -46.104) -> (-31.1486, -46.1044) construction
  line L229 (-31.1486, -46.1044) -> (-31.1883, -46.0784) construction
  spline S73 degree 3 poles (-31.1883, -46.0784) (-31.2584, -46.0325) (-31.2418, -45.994) (-31.1095, -45.8962) knots 0 0 0 0 1 1 1 1
  line L230 (-31.1883, -46.0784) -> (-31.2584, -46.0325) construction
  line L231 (-31.2584, -46.0325) -> (-31.2418, -45.994) construction
  line L232 (-31.2418, -45.994) -> (-31.1095, -45.8962) construction
  spline S74 degree 3 poles (-31.1095, -45.8962) (-30.457, -45.4136) (-27.043, -43.5255) (-26.2697, -43.2195) knots 0 0 0 0 1 1 1 1
  line L233 (-31.1095, -45.8962) -> (-30.457, -45.4136) construction